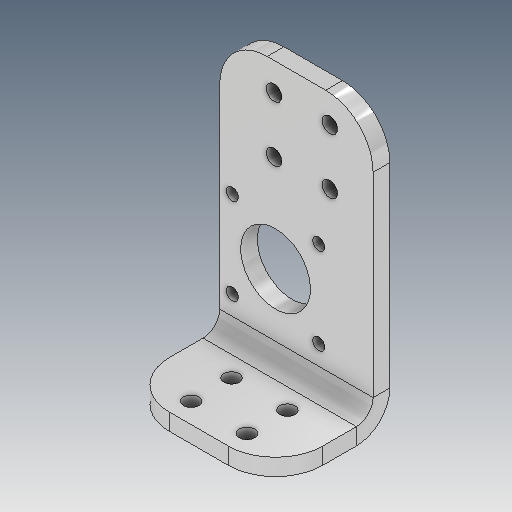
# Autodesk Inventor part: VerticalActuationPlate_V2
Saved by Autodesk Inventor 2020.3 (Build 243373000, 373)
## iProperties
Created: 2021-09-01
Part Number: VerticalActuationPlate_V2
Material: Aluminum 6061
Document SubType Name: Sheet Metal
Designer: justi
Density: 2.7 g/cm^3
Flat Pattern Width: 5.5 cm
Flat Pattern Length: 12.9572 cm
Flat Pattern Area: 71.2644 cm^2
Sheet Metal Rule: Default_mm
Sheet Metal Width: 55.000 mm
Sheet Metal Length: 129.572 mm
Sheet Metal Area: 7126.442 mm^2
Appearance: Aluminum - Polished
Mass: 99.9611 g
Surface Area: 160.122 cm^2
Volume: 37.0226 cm^3
Author: justi
Autodesk Inventor part; units mm, degrees
ref_plane "YZ Plane" through (0, 0, 0) normal (1, 0, 0) x (0, 1, 0)
ref_plane "XZ Plane" through (0, 0, 0) normal (0, 1, 0) x (-1, 0, 0)
ref_plane "XY Plane" through (0, 0, 0) normal (0, 0, 1) x (1, 0, 0)
sketch "Sketch2" plane through (0, 0, 0) normal (1, 0, 0) x (0, 1, 0)
  line L0 (43.5, 27.5) -> (-43.5, 27.5)
  line L1 (-43.5, 27.5) -> (-43.5, -27.5)
  line L2 (-43.5, -27.5) -> (43.5, -27.5)
  line L3 (43.5, -27.5) -> (43.5, 27.5)
  line L4 (43.5, 27.5) -> (-43.5, -27.5) construction
  line L5 (-43.5, 27.5) -> (43.5, -27.5) construction
  line L6 (-43.5, 27.5) -> (-21, 27.5) construction
  line L7 (-21, 27.5) -> (-21, 7.5) construction
  line L8 (-21, 7.5) -> (-43.5, 7.5) construction
  line L9 (-43.5, 7.5) -> (-43.5, 27.5) construction
  circle A0 centre (-21, 7.5) radius 12.5
  line L10 (-5.5, 23) -> (-36.5, 23) construction
  line L11 (-36.5, 23) -> (-36.5, -8) construction
  line L12 (-36.5, -8) -> (-5.5, -8) construction
  line L13 (-5.5, -8) -> (-5.5, 23) construction
  line L14 (-5.5, 23) -> (-36.5, -8) construction
  line L15 (-36.5, 23) -> (-5.5, -8) construction
  circle A1 centre (-5.5, 23) radius 2.15
  circle A2 centre (-5.5, -8) radius 2.15
  circle A3 centre (-36.5, 23) radius 2.15
  circle A4 centre (-36.5, -8) radius 2.15
  line L16 (43.5, -27.5) -> (23.5, -27.5) construction
  line L17 (23.5, -27.5) -> (23.5, -2) construction
  line L18 (23.5, -2) -> (43.5, -2) construction
  line L19 (43.5, -2) -> (43.5, -27.5) construction
  line L20 (33.5, 8) -> (13.5, 8) construction
  line L21 (13.5, 8) -> (13.5, -12) construction
  line L22 (13.5, -12) -> (33.5, -12) construction
  line L23 (33.5, -12) -> (33.5, 8) construction
  line L24 (33.5, 8) -> (13.5, -12) construction
  line L25 (13.5, 8) -> (33.5, -12) construction
  circle A5 centre (33.5, 8) radius 2.75
  circle A6 centre (33.5, -12) radius 2.75
  circle A7 centre (13.5, 8) radius 2.75
  circle A8 centre (13.5, -12) radius 2.75
  point P0 (0, 0)
  point P1 (0, 0)
  dimension "d47" = 24
  dimension "d20" = 87
  dimension "d21" = 55
  dimension "d22" = 22.5
  dimension "d23" = 20
  dimension "d24" = 25
  dimension "d25" = 31
  dimension "d26" = 31
  dimension "d27" = 4.3
  dimension "d28" = 4.3
  dimension "d29" = 4.3
  dimension "d30" = 4.3
  dimension "d31" = 20
  dimension "d32" = 25.5
  dimension "d33" = 20
  dimension "d34" = 20
  dimension "d35" = 5.5
  dimension "d36" = 5.5
  dimension "d37" = 5.5
  dimension "d38" = 5.5
extrude "Plate1" add sketch "Sketch2" along normal blind 6
sketch "Sketch3" plane through (12, -49.5, -27.5) normal (0, -1, 0) x (1, 0, 0)
  line L0 (0, 55) -> (0, 0)
  line L1 (0, 0) -> (29, 0)
  line L2 (29, 0) -> (29, 55)
  line L3 (29, 55) -> (0, 55)
  constraints: 6 end point, 1 horizontal, 1 perpendicular, 1 vertical
edge flange "Flange1" height 41 angle 90 thickness 6 bend radius 6 thickness toward (0, -1, 0) relief straight relief width 6 relief depth 3 edges at (6, -43.5, 0) wall of the first edge with corners at (12, -49.5, 27.5) (12, -49.5, -27.5) (41, -49.5, -27.5) (41, -49.5, 27.5)
bend "Bend1"
corner "Corner1"
sketch "Sketch4" plane through (41, -49.5, 27.5) normal (0, 1, 0) x (1, 0, 0)
  line L0 (-41, 16.75) -> (-41, 22.25) projected
  line L1 (-41, 17.5) -> (0, 17.5) construction
  line L2 (0, 0) -> (0, 55) projected
  line L3 (-35, 42.25) -> (-35, 36.75) projected
  line L4 (-35, 37.5) -> (0, 37.5) construction
  line L5 (0, 17.5) -> (-14.5, 17.5) construction
  line L6 (-20.5, 17.5) -> (-8.5, 17.5) construction
  line L7 (-24.286, 37.5) -> (-12.286, 37.5) construction
  line L8 (-14.5, 17.5) -> (-7.25, 17.5)
  line L9 (-14.5, 17.5) -> (-21.75, 17.5)
  circle A0 centre (-21.75, 17.5) radius 2.75
  circle A1 centre (-7.25, 17.5) radius 2.75
  line L10 (-14.5, 17.5) -> (-14.5, 37.5)
  line L11 (-14.5, 37.5) -> (-7.25, 37.5)
  line L12 (-14.5, 37.5) -> (-21.75, 37.5)
  circle A2 centre (-21.75, 37.5) radius 2.75
  circle A3 centre (-7.25, 37.5) radius 2.75
  line L13 (0, 27.5) -> (-14.5, 27.5)
  point P0 (-41, 27.5)
  point P1 (-14.5, 29.5)
  dimension "d50" = 14.5
  dimension "d58" = 7.25
  dimension "d59" = 7.25
  dimension "d60" = 5.5
  dimension "d61" = 5.5
  dimension "d62" = 7.25
  dimension "d63" = 7.25
  dimension "d64" = 5.5
  dimension "d65" = 5.5
  constraints: 26 end point, 5 point on line, 4 centre point, 4 coincident, 3 midpoint, 3 perpendicular, 1 horizontal
  measures "d50" distance of L1.end L5.end
  measures "d58" distance of L5.end L8.end
  measures "d59" distance of L5.end L9.end
  measures "d60" diameter of A0
  measures "d61" diameter of A1
  measures "d62" distance of L11.start L11.end
  measures "d63" distance of L11.start L12.end
  measures "d64" diameter of A2
  measures "d65" diameter of A3
extrude "Extrusion1" cut sketch "Sketch4" against normal through all
fillet "Fillet1" radius 17 4 edges at (3, 43.5, 27.5) (3, 43.5, -27.5) (41, -52.5, 27.5) (41, -52.5, -27.5)
equation "\"d47\" = CornerReliefSize"
equation "\"d39\" = Thickness"
equation "\"d40\" = BendReliefWidth"
equation "\"d41\" = BendReliefDepth"
equation "\"d42\" = MinimumRemnant"
equation "\"d43\" = TransitionRadius"
equation "\"d46\" = BendRadius"
equation "\"d48\" = GapSize"
equation "\"d49\" = JacobiRadiusSize"
equation "\"BendRadius\" = Thickness"
equation "\"BendReliefWidth\" = Thickness"
equation "\"BendReliefDepth\" = 0.5 * Thickness"
equation "\"CornerReliefSize\" = 4 * Thickness"
equation "\"MinimumRemnant\" = 2 * Thickness"
equation "\"TransitionRadius\" = BendRadius"
equation "\"JacobiRadiusSize\" = BendRadius"
equation "\"GapSize\" = Thickness"
equation "\"Thickness\" = 6"
body "Solid1"
